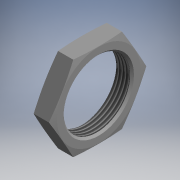
# Autodesk Inventor part: Flachmutter M20x1-5-24
Saved by Autodesk Inventor 2017.3 (Build 213256000, 256)
## iProperties
Part Number: Flachmutter M20x1-5-24
Material: Generic
Catalog Web Link: www.cadenas.de
Description: Thin nut-Thin nut
Vendor: FESTO
Document SubType Name: Modeling
Designer: partserver
Manufacturer: FESTO
Mass: 1.06017 g
Surface Area: 10.9151 cm^2
Volume: 1.06017 cm^3
Density: 1 g/cm^3
Appearance: PSOLRGB-175-175-175
Category: PARTsolutions
Company: FESTO
Title: Flachmutter M20x1-5-24
Author: Cadenas PARTsolutions
Comments: Thin nut
PSOL_IDENT_0: {$CADENAS_DATA\23d-libs\festo\zyl_zubeh\flachmuttern\thin_nut.prj},187 {VTYP=3D},{NB=Flachmutter M20
PSOL_IDENT_1: x1-5-24},{LINA=Flachmutter M20x1-5-24},{NN=Thin nut},{DATE=07.05.2020 13:37:03},{GEOMDATE=07.05.2020
PSOL_IDENT_2: 13:36:47},{VERSION=},{LINEID=390},{WBVAR=},{WBNUMERIC=}  {NB=Flachmutter M20x1-5-24},{LINA=Flachmut
PSOL_IDENT_3: ter M20x1-5-24},{KT=DUMMY},{TNR=},{TYP=Flachmutter},{D=M20x1},{DN=20.000},{D1=0.000},{H=5.000},{H1=0
PSOL_IDENT_4: .000},{SW=24.000},{P=1.000},{SCHL=M20x1-5-24},{VERS=1},{W=10.000}
NB: Flachmutter M20x1-5-24
NN: Thin nut
NT: Thin nut
NBSYN: $TYP. $SCHL.
LINA: Flachmutter M20x1-5-24
CATALOG: Festo
TYP: Flachmutter
D: M20x1
DN: 20
D1: 0
H: 5
H1: 0
SW: 24
P: 1
SCHL: M20x1-5-24
VERS: 1
W: 10
SUPPLIER: FESTO
ARTICLENO: Flachmutter M20x1-5-24
BOMINFO: Flachmutter M20x1-5-24
CREATOR: CADENAS GmbH
Autodesk Inventor part; units mm, degrees
ref_plane "YZ Plane" through (0, 0, 0) normal (1, 0, 0) x (0, 1, 0)
ref_plane "XZ Plane" through (0, 0, 0) normal (0, 1, 0) x (-1, 0, 0)
ref_plane "XY Plane" through (0, 0, 0) normal (0, 0, 1) x (1, 0, 0)
sketch "Skizze_1" plane through (0, 0, 0) normal (0, 0, 1) x (1, 0, 0)
  line L0 (5, 0) -> (0, 0)
  line L1 (0, 0) -> (0, 11.9)
  line L2 (0, 11.9) -> (0.864, 16.8)
  line L3 (0.864, 16.8) -> (4.136, 16.8)
  line L4 (4.136, 16.8) -> (5, 11.9)
  line L5 (5, 11.9) -> (5, 0)
  line L6 (5, 0) -> (0, 0)
  constraints: 14 end point
revolve "Revolution1" add sketch "Skizze_1" angle 360 about axis through (5, 0, 0) along (1, 0, 0)
sketch "Skizze_3" plane through (0, 0, 0) normal (0, 0, 1) x (1, 0, 0)
  line L0 (5, 0) -> (0, 0)
  line L1 (0, 0) -> (0, 10)
  line L2 (0, 10) -> (0.5415, 9.4585)
  line L3 (0.5415, 9.4585) -> (4.4585, 9.4585)
  line L4 (4.4585, 9.4585) -> (5, 10)
  line L5 (5, 10) -> (5, 0)
  line L6 (5, 0) -> (0, 0)
  constraints: 14 end point
revolve "Revolution2" cut sketch "Skizze_3" angle 360 about axis through (5, 0, 0) along (1, 0, 0)
thread "Thread1" size "M20x1" class "6H" standard "ISO Metric profile" full length
sketch "Sketch_1" plane through (0, 0, 0) normal (1, 0, 0) x (0, 1, 0)
  line L0 (24, 24) -> (-24, 24)
  line L1 (-24, 24) -> (-24, -24)
  line L2 (-24, -24) -> (24, -24)
  line L3 (24, -24) -> (24, 24)
  line L4 (-6.9282, 12) -> (-13.8564, 0)
  line L5 (-13.8564, 0) -> (-6.9282, -12)
  line L6 (-6.9282, -12) -> (6.9282, -12)
  line L7 (6.9282, -12) -> (13.8564, 0)
  line L8 (13.8564, 0) -> (6.9282, 12)
  line L9 (6.9282, 12) -> (-6.9282, 12)
  constraints: 20 end point
extrude "Extrusion1" cut sketch "Sketch_1" along normal blind 5
ref_plane "ANBAU_XY" through (0, 0, 0) normal (1, 0, 0) x (0, 0, -1)
ref_plane "ANBAU_YZ" through (0, 0, 0) normal (0, 0, -1) x (0, 1, 0)
ref_plane "ANBAU_ZX" through (0, 0, 0) normal (0, 1, 0) x (1, 0, 0)
ref_plane "SLE_XY" through (5, 0, 0) normal (-1, 0, 0) x (0, 1, 0)
ref_plane "SLE_YZ" through (5, 0, 0) normal (0, 1, 0) x (0, 0, -1)
ref_plane "SLE_ZX" through (5, 0, 0) normal (0, 0, -1) x (-1, 0, 0)
body "Solid1"
